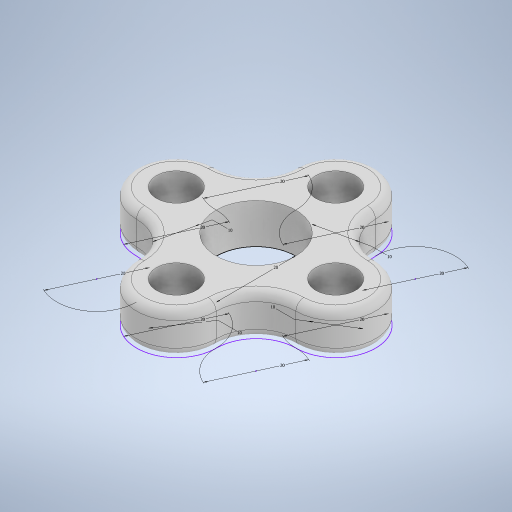
# Autodesk Inventor part: 孔2
Saved by Autodesk Inventor 2024.2 (Build 282272000, 272)
## iProperties
Created: 2024-03-28
Part Number: 孔2
Material: 一般
Document SubType Name: Modeling
Designer: User
Density: 1 g/cm^3
Appearance: 預設
Author: User
Autodesk Inventor part; units mm, degrees
ref_plane "YZ Plane" through (0, 0, 0) normal (1, 0, 0) x (0, 1, 0)
ref_plane "XZ Plane" through (0, 0, 0) normal (0, 1, 0) x (-1, 0, 0)
ref_plane "XY Plane" through (0, 0, 0) normal (0, 0, 1) x (1, 0, 0)
sketch "草圖1" plane through (0, 0, 0) normal (0, 1, 0) x (-1, 0, 0)
  point P0 (0, 0)
sketch "草圖2" plane through (0, 0, 0) normal (0, 1, 0) x (-1, 0, 0)
  circle A0 centre (0, 0) radius 10
  arc A1 (-10, -19.9999) -> (9.9999, -19.9545) centre (0, -20) ccw
  arc A2 (10, 20) -> (-10, 20) centre (0, 20) ccw
  arc A3 (-20, 10) -> (-19.9615, -9.9999) centre (-20, 0) ccw
  arc A4 (19.9614, -9.9999) -> (20, 10) centre (20, 0) ccw
  arc A5 (10, 20) -> (20, 10) centre (20, 20) ccw
  arc A6 (20.0384, -9.9999) -> (9.9999, -20.0453) centre (19.9998, -19.9999) ccw
  arc A7 (-10, -19.9999) -> (-20.0385, -9.9999) centre (-20, -19.9999) ccw
  arc A8 (-20, 10) -> (-10, 20) centre (-20, 20) ccw
  circle A9 centre (20, 0) radius 5
  circle A10 centre (0, -20) radius 5
  circle A11 centre (-20, 0) radius 5
  circle A12 centre (0, 20) radius 5
  dimension "d0" = 20
  dimension "d1" = 20
  dimension "d2" = 20
  dimension "d4" = 20
  dimension "d7" = 20
  dimension "d8" = 20
  dimension "d9" = 20
  dimension "d10" = 20
  dimension "d11" = 20
  dimension "d12" = 10
  dimension "d13" = 10
  dimension "d14" = 10
  dimension "d15" = 10
  constraints: 24 point on circle, 13 centre point, 9 equal radius, 5 coincident
  measures "d0" diameter of A0
  measures "d1" diameter of A1
  measures "d2" diameter of A2
  measures "d4" diameter of A3
  measures "d7" diameter of A4
  measures "d8" diameter of A5
  measures "d9" diameter of A6
  measures "d10" diameter of A7
  measures "d11" diameter of A8
  measures "d12" diameter of A9
  measures "d13" diameter of A10
  measures "d14" diameter of A11
  measures "d15" diameter of A12
extrude "擠出1" add sketch "草圖2" along normal blind 10
fillet "圓角1" radius 2 16 edges at (30, 10, 0.0193) (0, 10, 30) (-12.9289, 10, 12.9289) (-30, 10, 0.0192) (12.9289, 10, 12.9289) (12.9289, 0, 12.9289) (0, 0, 30) (-12.9289, 0, 12.9289) (-30, 0, 0.0192) (30, 0, 0.0193) (0.0227, 10, -30) (12.9425, 10, -12.9152) (12.9425, 0, -12.9152) (0.0227, 0, -30) (-12.9263, 10, -12.9312) (-12.9263, 0, -12.9312)
